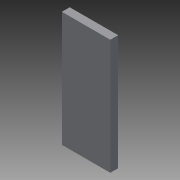
# Autodesk Inventor part: CNC-Z-axis- dremel mount backplate
Saved by Autodesk Inventor 2015 (Build 190159000, 159)
## iProperties
Created: 2015-03-21
Part Number: CNC-Z-axis- dremel mount backplate
Material: Generic
Document SubType Name: Modeling
Designer: Bangladesh
Density: 1 g/cm^3
Appearance: Default
Author: Bangladesh
Autodesk Inventor part; units mm, degrees
ref_plane "YZ Plane" through (0, 0, 0) normal (1, 0, 0) x (0, 1, 0)
ref_plane "XZ Plane" through (0, 0, 0) normal (0, 1, 0) x (-1, 0, 0)
ref_plane "XY Plane" through (0, 0, 0) normal (0, 0, 1) x (1, 0, 0)
sketch "Sketch1" plane through (0, 0, 0) normal (0, 0, 1) x (1, 0, 0)
  line L0 (-40, 95.16) -> (40, 95.16)
  line L1 (40, 95.16) -> (40, -95.16)
  line L2 (40, -95.16) -> (-40, -95.16)
  line L3 (-40, -95.16) -> (-40, 95.16)
  line L4 (-40, 95.16) -> (40, -95.16) construction
  line L5 (40, 95.16) -> (-40, -95.16) construction
  point P0 (0, 0)
  dimension "d0" = 80
  dimension "d1" = 190.32
  constraints: 12 end point, 2 midpoint, 2 parallel, 1 horizontal, 1 perpendicular
  measures "d0" distance of L1.end L2.end
  measures "d1" distance of L0.end L1.end
extrude "Extrusion1" add sketch "Sketch1" along normal mid plane 13
body "Solid1"
